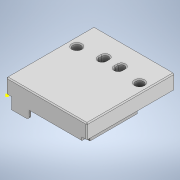
# Autodesk Inventor part: Cover_top
Saved by Autodesk Inventor 2022 (Build 260153000, 153)
## iProperties
Created: 2021-08-03
Part Number: Cover_top
Material: Generic
Document SubType Name: Modeling
Designer: exllu
Density: 1 g/cm^3
Appearance: Default
Author: exllu
Autodesk Inventor part; units mm, degrees
ref_plane "YZ Plane" through (0, 0, 0) normal (1, 0, 0) x (0, 1, 0)
ref_plane "XZ Plane" through (0, 0, 0) normal (0, 1, 0) x (-1, 0, 0)
ref_plane "XY Plane" through (0, 0, 0) normal (0, 0, 1) x (1, 0, 0)
sketch "Sketch1" plane through (0, 0, 0) normal (0, 1, 0) x (-1, 0, 0)
  line L0 (0, 0) -> (-80, 0)
  line L1 (-80, 0) -> (-80, -83)
  line L2 (-80, -83) -> (0, -83)
  line L3 (0, -83) -> (0, 0)
  dimension "d0" = 80
  dimension "d1" = 83
  constraints: 8 end point, 2 parallel, 1 horizontal, 1 perpendicular
  measures "d0" distance of L2.end L1.end
  measures "d1" distance of L1.end L0.end
extrude "Extrusion1" add sketch "Sketch1" along normal blind 16.25
sketch "Sketch2" plane through (0, 0, 0) normal (0, -1, 0) x (1, 0, 0)
  line L0 (0, -83) -> (0, 0) projected
  line L1 (0, 0) -> (0, -83)
  line L2 (80, -83) -> (0, -83) projected
  line L3 (80, 0) -> (80, -83) projected
  line L4 (0, -83) -> (80, -83)
  line L5 (80, -83) -> (80, -49.5)
  line L6 (80, -49.5) -> (0, -49.5)
  line L7 (0, -49.5) -> (0, -83)
  line L8 (80, -49.5) -> (0, -49.5)
  line L9 (0, -49.5) -> (0, 0)
  line L10 (0, 0) -> (80, 0)
  line L11 (80, 0) -> (80, -49.5)
  dimension "d4" = 33.5
  constraints: 18 end point, 4 parallel, 2 horizontal, 2 perpendicular, 1 point on line, 1 vertical
  measures "d4" distance of L5.end L4.end
extrude "Extrusion3" cut sketch "Sketch2" against normal blind 4 contours L0 L10 L3 L6
sketch "Sketch3" plane through (0, 4, 0) normal (0, -1, 0) x (1, 0, 0)
  line L0 (0, -83) -> (0, 0) projected
  line L1 (80, -49.5) -> (0, -49.5) projected
  line L2 (0, 0) -> (80, 0)
  line L3 (80, 0) -> (80, -49.5)
  line L4 (80, -49.5) -> (0, -49.5)
  line L5 (0, -49.5) -> (0, 0)
  constraints: 8 end point, 2 parallel, 1 horizontal, 1 perpendicular
extrude "Extrusion4" add sketch "Sketch3" along normal blind 13.169
sketch "Sketch4" plane through (0, 16.25, 0) normal (0, 0, 1) x (1, 0, 0)
  line L0 (80, 0) -> (0, 0) projected
  line L1 (0, 0) -> (80, 0)
  line L2 (80, -25.419) -> (80, 0) projected
  line L3 (80, 0) -> (80, -25.419)
  line L4 (80, -25.419) -> (38, -25.419)
  line L5 (80, -25.419) -> (0, -25.419) projected
  line L6 (38, -25.419) -> (38, -17)
  line L7 (38, -17) -> (80, -17)
  line L8 (80, -25.419) -> (77.5, -25.419)
  line L9 (77.5, -25.419) -> (77.5, -17)
  line L10 (77.5, -17) -> (80, -17)
  line L11 (77.5, -25.419) -> (75, -25.419)
  line L12 (75, -25.419) -> (75, -17)
  line L13 (75, -17) -> (77.5, -17)
  line L14 (77.5, -17) -> (77.5, -25.419)
  point P0 (0, -16.25)
  dimension "d11" = 42
  dimension "d12" = 8.419
  dimension "d13" = 2.5
  dimension "d14" = 2.5
  constraints: 24 end point, 6 perpendicular, 5 point on line, 2 horizontal, 2 parallel
  measures "d11" distance of L2.start L4.end
  measures "d12" distance of L4.end L6.end
  measures "d13" distance of L2.start L8.end
  measures "d14" distance of L12.end L13.end
extrude "Extrusion5" cut sketch "Sketch4" against normal blind 50 contours L4 L9 L7 L2 | L4 L6 L7 L12
sketch "Sketch5" plane through (77.5, -0.75, 0) normal (0, -1, 0) x (1, 0, 0)
  line L0 (-77.5, 0) -> (2.5, 0) projected
  line L1 (0, -49.5) -> (0, 0) projected
  line L2 (2.5, 0) -> (0, 0)
  line L3 (0, 0) -> (0, -49.5)
  line L4 (0, -49.5) -> (2.5, -49.5)
  line L5 (2.5, -49.5) -> (2.5, 0)
  constraints: 8 end point, 2 parallel, 1 horizontal, 1 perpendicular
extrude "Extrusion6" cut sketch "Sketch5" against normal blind 4.249
sketch "Sketch6" plane through (0, -9.169, 0) normal (0, -1, 0) x (1, 0, 0)
  line L0 (77.5, -49.5) -> (77.5, 0) projected
  line L1 (75, 0) -> (75, -49.5) projected
  line L2 (77.5, 0) -> (75, 0)
  line L3 (75, 0) -> (75, -2)
  line L4 (75, -2) -> (77.5, -2)
  line L5 (77.5, -2) -> (77.5, 0)
  point P0 (0, 0)
  dimension "d19" = 2
  constraints: 8 end point, 2 parallel, 1 horizontal, 1 perpendicular, 1 point on line
  measures "d19" distance of L3.end L2.end
extrude "Extrusion7" cut sketch "Sketch6" against normal blind 12.668
ref_plane "Work Plane1" through (40, 0, -83) normal (1, 0, 0) x (0, 0, -1)
mirror "Mirror1" about plane through (40, 0, -83) normal (1, 0, 0) of "Extrusion7", "Extrusion6"
sketch "Sketch7" plane through (0, -0.75, 0) normal (0, 0, 1) x (1, 0, 0)
  line L0 (0, 0) -> (0, -8.419) projected
  line L1 (2.5, -8.419) -> (0, -8.419) projected
  line L2 (0, 0) -> (2.5, 0)
  line L3 (2.5, 0) -> (2.5, -8.419)
  line L4 (2.5, -8.419) -> (0, -8.419)
  line L5 (0, -8.419) -> (0, 0)
  point P0 (0, 0.75)
  constraints: 8 end point, 2 parallel, 1 horizontal, 1 perpendicular
extrude "Extrusion8" cut sketch "Sketch7" against normal blind 50
sketch "Sketch8" plane through (0, -9.169, 0) normal (0, -1, 0) x (1, 0, 0)
  line L0 (2.5, -2) -> (5, -2) projected
  line L1 (75, -49.5) -> (38, -49.5) projected
  line L2 (5, -2) -> (75, -2)
  line L3 (75, -2) -> (75, -49.5)
  line L4 (75, -49.5) -> (5, -49.5)
  line L5 (5, -49.5) -> (5, -2)
  point P0 (0, 0)
  constraints: 8 end point, 2 parallel, 1 horizontal, 1 perpendicular
extrude "Extrusion9" cut sketch "Sketch8" against normal blind 22.419
sketch "Sketch10" plane through (0, 0, -83) normal (-1, 0, 0) x (0, 0, 1)
  line L0 (0, 0) -> (0, 16.25) projected
  line L1 (33.5, 0) -> (33.5, 13.25) projected
  line L2 (0, 0) -> (33.5, 0)
  line L3 (33.5, 0) -> (33.5, 3.5)
  line L4 (33.5, 3.5) -> (0, 3.5)
  line L5 (0, 3.5) -> (0, 0)
  point P0 (83, 0)
  dimension "d30" = 3.5
  constraints: 8 end point, 2 parallel, 1 horizontal, 1 perpendicular, 1 point on line
  measures "d30" distance of L3.end L2.end
extrude "Extrusion11" cut sketch "Sketch10" against normal blind 5.5
mirror "Mirror2" about plane through (40, 0, -83) normal (1, 0, 0) of "Extrusion11"
sketch "Sketch11" plane through (80, 16.25, -83) normal (0, 0, -1) x (-1, 0, 0)
  line L0 (80, -16.25) -> (64.5, -16.25)
  line L1 (5.5, -16.25) -> (74.5, -16.25) projected
  line L2 (64.5, -16.25) -> (64.5, -12.75)
  line L3 (64.5, -16.25) -> (68, -16.25) construction
  line L4 (74.5, -12.75) -> (80, -12.75) projected
  line L5 (64.5, -12.75) -> (74.5, -12.75)
  line L6 (74.5, -16.25) -> (74.5, -12.75) projected
  line L7 (74.5, -12.75) -> (74.5, -16.25)
  dimension "d33" = 15.5
  dimension "d34" = 3.5
  dimension "d35" = 90
  constraints: 10 end point, 2 perpendicular, 1 collinear, 1 horizontal, 1 point on line
  measures "d33" distance of L0.start L0.end
  measures "d34" distance of L0.end L2.end
  measures "d35" angle of L3 L2
extrude "Extrusion12" cut sketch "Sketch11" against normal blind 3.5
sketch "Sketch12" plane through (74.5, 3.5, -83) normal (0, -1, 0) x (1, 0, 0)
  line L0 (0, 0) -> (-59, 0) projected
  line L1 (5.5, 83) -> (5.5, 0) projected
  line L2 (0, 0) -> (5.5, 0)
  line L3 (5.5, 0) -> (5.5, 2.5)
  line L4 (5.5, 2.5) -> (0, 2.5)
  line L5 (0, 2.5) -> (0, 0)
  point P0 (-74.5, 83)
  dimension "d38" = 2.5
  constraints: 8 end point, 2 parallel, 1 horizontal, 1 perpendicular, 1 point on line
  measures "d38" distance of L3.end L2.end
extrude "Extrusion13" add sketch "Sketch12" along normal blind 3.5
sketch "Sketch13" plane through (0, 0, 0) normal (0, -1, 0) x (1, 0, 0)
  line L0 (80, 0) -> (80, -83) projected
  line L1 (80, -83) -> (65, -83)
  line L2 (65, -83) -> (65, -80.5)
  line L3 (65, -80.5) -> (80, -80.5)
  line L4 (80, -80.5) -> (80, -83)
  point P0 (0, 0)
  dimension "d41" = 15
  dimension "d42" = 2.5
  constraints: 8 end point, 2 parallel, 1 horizontal, 1 perpendicular
  measures "d41" distance of L2.end L3.end
  measures "d42" distance of L1.end L2.end
extrude "Extrusion14" add sketch "Sketch13" along normal blind 16.831
sketch "Sketch15" plane through (0, 16.25, 0) normal (0, 1, 0) x (1, 0, 0)
  line L0 (0, 0) -> (0, 83)
  line L1 (65, 83) -> (15.5, 83) projected
  line L2 (0, 83) -> (80, 83)
  line L3 (40, 83) -> (40, 60)
  line L4 (40, 60) -> (48, 60)
  line L5 (48, 60) -> (32, 60)
  circle A0 centre (32, 60) radius 1.75
  circle A1 centre (48, 60) radius 1.75
  dimension "d55" = 83
  dimension "d57" = 80
  dimension "d58" = 23
  dimension "d59" = 8
  dimension "d60" = 16
  dimension "d61" = 3.5
  dimension "d62" = 3.5
  constraints: 10 end point, 2 centre point, 2 coincident, 2 point on line, 2 vertical, 1 horizontal, 1 midpoint
  measures "d55" distance of L0.start L0.end
  measures "d57" distance of L0.end L2.end
  measures "d58" distance of L3.start L3.end
  measures "d59" distance of L3.end L4.end
  measures "d60" distance of L4.end L5.end
  measures "d61" diameter of A0
  measures "d62" diameter of A1
extrude "Extrusion16" cut sketch "Sketch15" against normal blind 50
sketch "Sketch16" plane through (0, 16.25, 0) normal (0, 1, 0) x (1, 0, 0)
  circle A0 centre (32, 60) radius 1.75 projected
  circle A1 centre (32, 60) radius 4
  circle A2 centre (48, 60) radius 1.75 projected
  circle A3 centre (48, 60) radius 4
  point P0 (0, 0)
  dimension "d65" = 8
  dimension "d66" = 8
  constraints: 2 centre point, 2 coincident
  measures "d65" diameter of A1
  measures "d66" diameter of A3
extrude "Extrusion17" cut sketch "Sketch16" against normal blind 10
sketch "Sketch19" plane through (0, 0, 0) normal (0, -1, 0) x (1, 0, 0)
  line L0 (74.5, -80.5) -> (74.5, -49.5) projected
  line L1 (15.5, -79.5) -> (5.5, -79.5) projected
  line L2 (74.5, -49.5) -> (5.5, -49.5)
  line L3 (5.5, -49.5) -> (5.5, -79.5)
  line L4 (5.5, -79.5) -> (15.5, -79.5)
  line L5 (74.5, -79.5) -> (74.5, -49.5)
  line L6 (15.5, -83) -> (15.5, -79.5) projected
  line L7 (65, -80.5) -> (65, -83) projected
  line L8 (15.5, -79.5) -> (65, -79.5)
  line L9 (65, -80.5) -> (65, -83)
  line L10 (65, -83) -> (15.5, -83)
  line L11 (15.5, -83) -> (15.5, -79.5)
  line L12 (65, -80.5) -> (74.5, -80.5) projected
  line L13 (74.5, -79.5) -> (65, -79.5)
  line L14 (65, -79.5) -> (65, -80.5)
  line L15 (65, -80.5) -> (74.5, -80.5)
  line L16 (74.5, -80.5) -> (74.5, -79.5)
  point P0 (0, 0)
  constraints: 24 end point, 6 parallel, 3 horizontal, 3 perpendicular, 2 point on line
extrude "Extrusion20" cut sketch "Sketch19" against normal blind 1.25
sketch "Sketch20" plane through (0, -9.169, 0) normal (0, -1, 0) x (1, 0, 0)
  line L0 (0, -49.5) -> (5, -49.5) projected
  line L1 (2.5, -2) -> (2.5, -49.5) projected
  line L2 (5, -49.5) -> (2.5, -49.5)
  line L3 (2.5, -49.5) -> (2.5, -2)
  line L4 (2.5, -2) -> (5, -2)
  line L5 (5, -2) -> (5, -49.5)
  line L6 (5, -2) -> (2.5, -2) projected
  line L7 (5, -2) -> (5.9402, -2)
  line L8 (5.9402, -2) -> (5.9402, -3.7491)
  line L9 (5.9402, -3.7491) -> (5, -3.7491)
  line L10 (5, -3.7491) -> (5, -2)
  point P0 (0, 0)
  constraints: 16 end point, 4 parallel, 2 horizontal, 2 perpendicular
extrude "Extrusion21" cut sketch "Sketch20" against normal blind 6
mirror "Mirror5" about plane through (40, 0, -83) normal (1, 0, 0) of "Extrusion21"
sketch "Sketch21" plane through (77.5, 3.499, -2) normal (1, 0, 0) x (0, 0, -1)
  line L0 (0, -6.668) -> (0, 0) projected
  line L1 (0, -6.668) -> (47.5, -6.668) projected
  line L2 (0, 0) -> (47.5, 0)
  line L3 (47.5, 0) -> (47.5, -6.668)
  line L4 (47.5, -6.668) -> (0, -6.668)
  line L5 (0, -6.668) -> (0, 0)
  point P0 (-2, -3.499)
  point P1 (1, -6.668)
  constraints: 8 end point, 2 parallel, 1 horizontal, 1 perpendicular
extrude "Extrusion22" cut sketch "Sketch21" against normal blind 0.5
mirror "Mirror6" about plane through (40, 0, -83) normal (1, 0, 0) of "Extrusion22"
sketch "Sketch22" plane through (5, -3.169, -2) normal (0, 0, 1) x (1, 0, 0)
  line L0 (0, 0) -> (-2, 0) projected
  line L1 (-5, 6.668) -> (0, 6.668) projected
  line L2 (0, 0) -> (-2, 0)
  line L3 (-2, 0) -> (-2, 6.668)
  line L4 (-2, 6.668) -> (0, 6.668)
  line L5 (0, 6.668) -> (0, 0)
  point P0 (-5, 3.169)
  point P1 (-4, 6.668)
  constraints: 8 end point, 2 parallel, 1 horizontal, 1 perpendicular, 1 point on line
extrude "Extrusion23" cut sketch "Sketch22" against normal blind 1
mirror "Mirror7" about plane through (40, 0, -83) normal (1, 0, 0) of "Extrusion23"
sketch "Sketch23" plane through (0, 16.25, 0) normal (0, 1, 0) x (1, 0, 0)
  circle A0 centre (32, 60) radius 4 projected
  arc A1 (36, 60) -> (28, 60) centre (32, 60) ccw
  line L0 (32, 60) -> (32, 57)
  arc A2 (28, 57) -> (36, 57) centre (32, 57) ccw
  line L1 (28, 57) -> (28, 60)
  line L2 (36, 60) -> (36, 57)
  line L3 (79, 83) -> (1, 83) projected
  line L4 (1, 83) -> (79, 83)
  line L5 (1, 83) -> (40, 83)
  line L6 (40, 83) -> (40, 30.6783)
  line L7 (65, 83) -> (80, 83) projected
  circle A3 centre (48, 60) radius 4
  arc A4 (52, 60) -> (44, 60) centre (48, 60) ccw
  line L8 (48, 60) -> (48, 57)
  arc A5 (44, 57) -> (52, 57) centre (48, 57) ccw
  line L9 (52, 57) -> (52, 60)
  line L10 (44, 60) -> (44, 57)
  point P0 (0, 0)
  point P1 (52, 60)
  point P2 (44, 60)
  dimension "d87" = 8
  dimension "d88" = 3
  dimension "d89" = 8
  dimension "d90" = 39
  constraints: 18 end point, 8 point on circle, 8 symmetric about line, 5 centre point, 4 coincident, 3 tangent, 1 collinear, 1 midpoint, 1 perpendicular, 1 vertical, 3 other
  measures "d87" diameter of A1
  measures "d88" distance of L0.start L0.end
  measures "d89" diameter of A2
  measures "d90" distance of L3.end L5.end
sketch "Sketch24" plane through (0, 6.25, 0) normal (0, 1, 0) x (1, 0, 0)
  arc A0 (33.75, 60) -> (30.25, 60) centre (32, 60) ccw
  circle A1 centre (48, 60) radius 1.75 projected
  arc A2 (49.75, 60) -> (46.25, 60) centre (48, 60) ccw
  line L0 (48, 60) -> (48, 57)
  arc A3 (46.25, 57) -> (49.75, 57) centre (48, 57) ccw
  line L1 (46.25, 57) -> (46.25, 60)
  line L2 (49.75, 60) -> (49.75, 57)
  circle A4 centre (32, 60) radius 1.75 projected
  line L3 (32, 60) -> (32, 63)
  arc A5 (36, 63) -> (28, 63) centre (32, 63) ccw
  circle A6 centre (32, 60) radius 4 projected
  line L4 (28, 60) -> (28, 63)
  line L5 (36, 63) -> (36, 60)
  arc A7 (28, 60) -> (36, 60) centre (32, 60) ccw
  line L6 (32, 60) -> (48, 60)
  line L7 (40, 60) -> (40, 64.9019)
  arc A8 (52, 63) -> (44, 63) centre (48, 63) ccw
  line L8 (52, 60) -> (52, 63)
  line L9 (44, 63) -> (44, 60)
  arc A9 (44, 60) -> (52, 60) centre (48, 60) ccw
  point P0 (0, 0)
  point P1 (49.75, 60)
  point P2 (46.25, 60)
  point P3 (49.6223, 56.3437)
  point P4 (46.25, 60)
  dimension "d93" = 3.5
  dimension "d94" = 3.5
  dimension "d96" = 3
  dimension "d98" = 3.5
  dimension "d107" = 3
  dimension "d108" = 8
  constraints: 20 end point, 16 point on circle, 7 centre point, 6 symmetric about line, 6 tangent, 5 coincident, 3 vertical, 1 horizontal, 1 midpoint, 2 other
  measures "d93" diameter of A0
  measures "d94" diameter of A2
  measures "d96" distance of L0.start L0.end
  measures "d98" diameter of A3
  measures "d107" distance of L3.start L3.end
  measures "d108" diameter of A5
sketch "Sketch25" plane through (0, 1.25, 0) normal (0, -1, 0) x (1, 0, 0)
  line L0 (0, -49.5) -> (5, -49.5) projected
  line L1 (0, 0) -> (0, -49.5)
  line L2 (5.5, -49.5) -> (74.5, -49.5) projected
  line L3 (0, -49.5) -> (5.5, -49.5)
  line L4 (5.5, -79.5) -> (5.5, -49.5) projected
  circle A0 centre (71, -55) radius 4 projected
  line L5 (5.5, -49.5) -> (74.1225, -49.5)
  line L6 (74.1225, -49.5) -> (74.1225, -52.5)
  line L7 (74.1225, -52.5) -> (5.5, -52.5)
  line L8 (5.5, -52.5) -> (5.5, -49.5)
  dimension "d104" = 3
  constraints: 12 end point, 2 parallel, 1 collinear, 1 horizontal, 1 perpendicular, 1 vertical, 2 other
  measures "d104" distance of L5.end L6.end
extrude "Extrusion26" cut sketch "Sketch25" against normal blind 12 contours L2 L6 A0 L7 L4 | L7 A0 picked at (71, -52)
extrude "Extrusion27" cut sketch "Sketch24" along normal blind 12 contours A1 L6 L9 A8 L8 A9 A3 L2 | L5 A6 L4 A5
sketch "Sketch26" plane through (0, 6.25, 0) normal (0, 1, 0) x (1, 0, 0)
  circle A0 centre (32, 60) radius 1.75 projected
  line L0 (32, 60) -> (32, 63)
  circle A1 centre (48, 60) radius 1.75 projected
  line L1 (48, 60) -> (48, 63)
  circle A2 centre (48, 63) radius 1.75
  arc A3 (33.75, 63) -> (30.25, 63) centre (32, 63) ccw
  line L2 (30.25, 63) -> (30.25, 60)
  line L3 (46.25, 63) -> (46.25, 60)
  line L4 (33.75, 63) -> (33.75, 60)
  arc A4 (30.25, 60) -> (33.75, 60) centre (32, 60) ccw
  line L5 (32, 60) -> (48, 60)
  line L6 (40, 60) -> (40, 64.1787)
  circle A5 centre (48, 60) radius 1.75
  arc A6 (49.75, 63) -> (46.25, 63) centre (48, 63) ccw
  line L7 (49.75, 63) -> (49.75, 60)
  line L8 (46.25, 63) -> (46.25, 60)
  point P0 (0, 0)
  point P1 (47.0986, 61.5)
  point P2 (48.9014, 61.5)
  point P3 (49.75, 60)
  dimension "d113" = 3.5
  dimension "d111" = 3
  dimension "d112" = 3
  dimension "d114" = 3.5
  constraints: 18 end point, 10 point on circle, 4 centre point, 4 symmetric about line, 4 tangent, 4 vertical, 3 coincident, 1 midpoint, 1 perpendicular, 7 other
  measures "d111" distance of L0.start L0.end
  measures "d112" distance of L1.start L1.end
  measures "d114" diameter of A3
extrude "Extrusion28" cut sketch "Sketch26" against normal blind 12 contours L2 A3 L4 A0 | L3 A2 A1 | A1 A2 L7 | A2 A1 | A1 L1 A2 | A2 L1 A1
sketch "Sketch29" plane through (0, 16.25, 0) normal (0, 1, 0) x (1, 0, 0)
  arc A0 (72.75, 58) -> (69.25, 58) centre (71, 58) ccw projected
  circle A1 centre (71, 58) radius 1.75
  point P0 (0, 0)
  constraints: 1 centre point, 1 coincident
extrude "Extrusion30" cut sketch "Sketch29" against normal blind 30
sketch "Sketch30" plane through (0, 16.25, 0) normal (0, 1, 0) x (1, 0, 0)
  circle A0 centre (71, 58) radius 1.75 projected
  circle A1 centre (71, 58) radius 4
  point P0 (0, 0)
  dimension "d129" = 8
  constraints: 1 centre point, 1 coincident
  measures "d129" diameter of A1
extrude "Extrusion31" cut sketch "Sketch30" against normal blind 12 contours A0 | A1
mirror "Mirror8" about plane through (40, 0, -83) normal (1, 0, 0) of "Extrusion30", "Extrusion31"
sketch "Sketch31" plane through (74.5, 3.5, -49.5) normal (1, 0, 0) x (0, 0, -1)
  line L0 (3, 0) -> (0, 0) projected
  line L1 (3, -2.25) -> (3, 0) projected
  line L2 (0, 0) -> (3, 0)
  line L3 (3, 0) -> (3, -2.25)
  line L4 (3, -2.25) -> (0, -2.25)
  line L5 (0, -2.25) -> (0, 0)
  point P0 (-49.5, -3.5)
  constraints: 8 end point, 2 parallel, 1 horizontal, 1 perpendicular
extrude "Extrusion32" cut sketch "Sketch31" against normal blind 100
sketch "Sketch32" plane through (0, 16.25, 0) normal (0, 0, 1) x (1, 0, 0)
  line L0 (0, -12.751) -> (0, 0) projected
  line L1 (80, -12.751) -> (80, 0) projected
  line L2 (0, 0) -> (80, 0)
  line L3 (80, 0) -> (80, -12.751)
  line L4 (80, -12.751) -> (75, -12.751)
  line L5 (75, -17) -> (75, -12.751) projected
  line L6 (75, -12.751) -> (75, -17)
  line L7 (38, -17) -> (75, -17) projected
  line L8 (75, -17) -> (38, -17)
  line L9 (38, -25.419) -> (5, -25.419) projected
  line L10 (38, -17) -> (38, -25.419)
  line L11 (38, -25.419) -> (5, -25.419)
  line L12 (5, -12.751) -> (5, -25.419) projected
  line L13 (5, -25.419) -> (5, -12.751)
  line L14 (0, -12.751) -> (5, -12.751) projected
  line L15 (5, -12.751) -> (0, -12.751)
  line L16 (0, -12.751) -> (0, 0)
  point P0 (0, -16.25)
  constraints: 20 end point, 5 perpendicular, 4 collinear, 1 horizontal
extrude "Extrusion33" add sketch "Sketch32" along normal blind 2
sketch "Sketch33" plane through (38, -9.169, -2) normal (0, 0, -1) x (-1, 0, 0)
  line L0 (0, 0) -> (0, 8.419) projected
  line L1 (33, 0) -> (0, 0) projected
  line L2 (0, 0) -> (33, 0)
  line L3 (33, 12.668) -> (33, 22.419) projected
  line L4 (33, 0) -> (33, 22.419)
  line L5 (33, 22.419) -> (-37, 22.419) projected
  line L6 (33, 22.419) -> (-37, 22.419)
  line L7 (-37, 8.419) -> (-37, 12.668) projected
  line L8 (-37, 22.419) -> (-37, 8.419)
  line L9 (0, 8.419) -> (-37, 8.419) projected
  line L10 (-37, 8.419) -> (0, 8.419)
  line L11 (0, 8.419) -> (0, 0)
  point P0 (38, 9.169)
  constraints: 12 end point, 3 collinear, 2 perpendicular, 1 horizontal
extrude "Extrusion34" cut sketch "Sketch33" against normal blind 2
sketch "Sketch35" plane through (74.1225, 3.5, -49.5) normal (-1, 0, 0) x (0, 0, 1)
  line L0 (0, -6.669) -> (0, 0) projected
  line L1 (-3, -2.25) -> (-3, 9.75) projected
  line L2 (0, 0) -> (-3, 0)
  line L3 (-3, 0) -> (-3, 9.75)
  line L4 (-3, 9.75) -> (0, 9.75)
  line L5 (0, 9.75) -> (0, 0)
  point P0 (49.5, -3.5)
  point P1 (-3, 0)
  point P2 (-3, 0)
  constraints: 8 end point, 2 parallel, 1 horizontal, 1 perpendicular
extrude "Extrusion36" cut sketch "Sketch35" against normal blind 0.878
sketch "Sketch36" plane through (5.5, 3.5, -52.5) normal (1, 0, 0) x (0, 0, -1)
  line L0 (0, 0) -> (-3, 0) projected
  line L1 (0, 0) -> (-3, 0)
  line L2 (-3, 0) -> (-3, 9.75)
  line L3 (-3, 9.75) -> (0, 9.75)
  line L4 (0, 9.75) -> (0, 0)
  point P0 (-52.5, -3.5)
  constraints: 8 end point, 2 parallel, 1 horizontal, 1 perpendicular
extrude "Extrusion37" cut sketch "Sketch36" against normal blind 0.5
sketch "Sketch37" plane through (0, 3.5, -83) normal (0, -1, 0) x (1, 0, 0)
  line L0 (80, 0) -> (0, 0) projected
  line L1 (15.5, 3.5) -> (5.5, 3.5) projected
  line L2 (0, 0) -> (15.5, 0)
  line L3 (15.5, 0) -> (15.5, 3.5)
  line L4 (15.5, 3.5) -> (0, 3.5)
  line L5 (0, 3.5) -> (0, 0)
  line L6 (0, 0) -> (5.5, 0)
  line L7 (5.5, 0) -> (5.5, 30.5)
  line L8 (5.5, 30.5) -> (0, 30.5)
  line L9 (0, 30.5) -> (0, 0)
  line L10 (5, 33.5) -> (3, 33.5) projected
  line L11 (0, 30.5) -> (5, 30.5)
  line L12 (5, 30.5) -> (5, 33.5)
  line L13 (5, 33.5) -> (0, 33.5)
  line L14 (0, 33.5) -> (0, 30.5)
  line L15 (0, 33.5) -> (0, 85) projected
  line L16 (0, 33.5) -> (0, 85)
  line L17 (0, 85) -> (5, 85)
  line L18 (80, 85) -> (0, 85) projected
  line L19 (5, 83) -> (5, 80) projected
  line L20 (5, 80) -> (5, 85)
  line L21 (3, 80) -> (5, 80) projected
  line L22 (5, 80) -> (3, 80)
  line L23 (3, 80) -> (3, 33.5) projected
  line L24 (3, 80) -> (3, 33.5)
  point P0 (0, 83)
  constraints: 34 end point, 6 parallel, 3 collinear, 3 horizontal, 3 perpendicular, 1 point on line, 1 vertical
extrude "Extrusion38" add sketch "Sketch37" along normal blind 1.25
sketch "Sketch38" plane through (74.5, 3.5, -80.5) normal (0, -1, 0) x (1, 0, 0)
  line L0 (5.5, 0) -> (-9.5, 0) projected
  line L1 (5.5, 82.5) -> (5.5, 31) projected
  line L2 (5.5, 0) -> (5.5, 82.5)
  line L3 (5.5, 82.5) -> (0.5, 82.5)
  line L4 (0.5, 82.5) -> (0.5, 77.5)
  line L5 (0.5, 80.5) -> (0.5, 31) projected
  line L6 (2.5, 77.5) -> (2.5, 31) projected
  line L7 (0.5, 77.5) -> (2.5, 77.5)
  line L8 (2.5, 77.5) -> (2.5, 31)
  line L9 (2.5, 31) -> (0.5, 31)
  line L10 (0.5, 31) -> (0.5, 28)
  line L11 (0.5, 28) -> (0, 28)
  line L12 (0.5005, 28) -> (-69.5, 28) projected
  line L13 (0, 28) -> (0, 0)
  line L14 (0, 0) -> (5.5, 0)
  point P0 (-74.5, 80.5)
  point P1 (0, 0)
  dimension "d151" = 5
  dimension "d152" = 0.5
  constraints: 20 end point, 4 perpendicular, 4 point on line, 2 collinear
  measures "d151" distance of L3.end L4.end
  measures "d152" distance of L10.end L11.end
extrude "Extrusion39" add sketch "Sketch38" along normal blind 1.25 contours L0 L13 L11 L10 L9 L6 L7 L4 L3 L1 L2
sketch "Sketch39" plane through (0, 1.25, 0) normal (0, -1, 0) x (1, 0, 0)
  line L0 (74.5, -80.5) -> (74.5, -52.5) projected
  line L1 (5.5, -52.5) -> (5.5, -79.5) projected
  line L2 (74.5, -80.5) -> (5.5, -80.5)
  line L3 (5.5, -80.5) -> (5.5, -52.5)
  line L4 (5.5, -52.5) -> (74.5, -52.5)
  line L5 (74.5, -52.5) -> (74.5, -80.5)
  line L6 (5.5, -79.5) -> (5.5, -52.5) projected
  line L7 (15.5, -83) -> (15.5, -79.5) projected
  line L8 (5.5, -79.5) -> (15.5, -79.5)
  line L9 (15.5, -79.5) -> (15.5, -80.5)
  line L10 (15.5, -80.5) -> (5.5, -80.5)
  line L11 (5.5, -80.5) -> (5.5, -79.5)
  line L12 (74.5, -80.5) -> (65, -80.5) projected
  line L13 (15.5, -83) -> (65, -83)
  line L14 (65, -83) -> (65, -80.5)
  line L15 (65, -80.5) -> (15.5, -80.5)
  line L16 (15.5, -80.5) -> (15.5, -83)
  point P0 (0, 0)
  constraints: 24 end point, 6 parallel, 3 horizontal, 3 perpendicular, 2 point on line
extrude "Extrusion40" add sketch "Sketch39" along normal blind 1.25 contours L2 L7 L8 L1 L4 L0 | L14 L13 L7 L2
sketch "Sketch40" plane through (0, 16.25, 0) normal (0, 1, 0) x (1, 0, 0)
  circle A0 centre (9, 58) radius 1.75 projected
  circle A1 centre (9, 58) radius 1.75
  circle A2 centre (9, 58) radius 4
  arc A3 (30.25, 60) -> (33.75, 60) centre (32, 60) ccw projected
  arc A4 (30.25, 60) -> (33.75, 60) centre (32, 60) ccw
  arc A5 (33.75, 63) -> (30.25, 63) centre (32, 63) ccw projected
  arc A6 (33.75, 63) -> (30.3777, 63.6563) centre (32, 63) ccw
  arc A7 (28, 60) -> (36, 60) centre (32, 60) ccw projected
  line L0 (36, 60) -> (36, 63)
  line L1 (33.75, 60) -> (33.75, 63) projected
  line L2 (33.75, 63) -> (33.75, 60)
  arc A8 (36, 63) -> (33.75, 66.5969) centre (32, 63) ccw
  arc A9 (28, 60) -> (36, 60) centre (32, 60) ccw
  arc A10 (36, 63) -> (28, 63) centre (32, 63) ccw
  line L3 (28, 60) -> (28, 63) projected
  line L4 (28, 60) -> (28, 63)
  line L5 (30.25, 63) -> (30.25, 60) projected
  line L6 (30.25, 60) -> (30.25, 63)
  arc A11 (46.25, 60) -> (49.75, 60) centre (48, 60) ccw projected
  line L7 (32, 60) -> (48, 60)
  line L8 (48, 60) -> (40, 60)
  line L9 (40, 60) -> (40, 47.3434)
  circle A12 centre (71, 58) radius 1.75
  circle A13 centre (71, 58) radius 1.75
  circle A14 centre (71, 58) radius 4
  arc A15 (46.25, 60) -> (49.75, 60) centre (48, 60) ccw
  arc A16 (46.25, 60) -> (49.75, 60) centre (48, 60) ccw
  arc A17 (49.75, 63) -> (46.25, 63) centre (48, 63) ccw
  arc A18 (49.6223, 63.6563) -> (46.25, 63) centre (48, 63) ccw
  arc A19 (44, 60) -> (52, 60) centre (48, 60) ccw
  line L10 (44, 60) -> (44, 63)
  line L11 (46.25, 60) -> (46.25, 63)
  line L12 (46.25, 63) -> (46.25, 60)
  arc A20 (46.25, 66.5969) -> (44, 63) centre (48, 63) ccw
  arc A21 (44, 60) -> (52, 60) centre (48, 60) ccw
  arc A22 (52, 63) -> (44, 63) centre (48, 63) ccw
  line L13 (52, 60) -> (52, 63)
  line L14 (52, 60) -> (52, 63)
  line L15 (49.75, 63) -> (49.75, 60)
  line L16 (49.75, 60) -> (49.75, 63)
  point P0 (0, 0)
  constraints: 30 point on circle, 28 end point, 23 symmetric about line, 18 centre point, 14 coincident, 4 point on line, 4 tangent, 2 collinear, 2 vertical, 1 horizontal, 1 midpoint, 11 other
extrude "Extrusion41" cut sketch "Sketch40" against normal blind 30 contours A0 | L5 A5 L1 A3 | L11 A17 L15 A11 | A12
sketch "Sketch41" plane through (0, 6.25, 0) normal (0, 1, 0) x (1, 0, 0)
  arc A0 (28, 60) -> (36, 60) centre (32, 60) ccw projected
  arc A1 (28, 60) -> (36, 60) centre (32, 60) ccw
  arc A2 (36, 63) -> (28, 63) centre (32, 63) ccw projected
  arc A3 (36, 63) -> (28, 63) centre (32, 63) ccw
  line L0 (28, 63) -> (28, 60) projected
  line L1 (28, 60) -> (28, 63)
  line L2 (36, 63) -> (37, 63) projected
  line L3 (36, 63) -> (36, 60)
  arc A4 (52, 63) -> (44, 63) centre (48, 63) ccw projected
  line L4 (32, 63) -> (48, 63)
  line L5 (40, 63) -> (40, 64.9814)
  arc A5 (44, 60) -> (52, 60) centre (48, 60) ccw
  arc A6 (44, 60) -> (52, 60) centre (48, 60) ccw
  arc A7 (52, 63) -> (44, 63) centre (48, 63) ccw
  arc A8 (52, 63) -> (44, 63) centre (48, 63) ccw
  line L6 (52, 63) -> (52, 60)
  line L7 (52, 60) -> (52, 63)
  line L8 (44, 63) -> (43, 63)
  line L9 (44, 63) -> (44, 60)
  line L10 (48, 63) -> (32, 63)
  point P0 (0, 0)
  constraints: 18 end point, 14 symmetric about line, 12 point on circle, 6 centre point, 6 point on line, 4 coincident, 1 collinear, 1 horizontal, 1 midpoint, 1 tangent, 1 vertical, 4 other
extrude "Extrusion42" cut sketch "Sketch41" against normal blind 4.25
sketch "Sketch42" plane through (65, -16.831, -80.5) normal (0, 0, 1) x (1, 0, 0)
  line L0 (0, 0) -> (0, 16.831) projected
  line L1 (15, 0) -> (0, 0) projected
  line L2 (0, 16.831) -> (15, 16.831)
  line L3 (15, 16.831) -> (15, 0)
  line L4 (15, 0) -> (0, 0)
  line L5 (0, 0) -> (0, 16.831)
  line L6 (15, 19.081) -> (9.5, 19.081) projected
  line L7 (9.5, 19.081) -> (15, 19.081)
  line L8 (15, 19.081) -> (15, 16.831)
  line L9 (15, 16.831) -> (9.5, 16.831)
  line L10 (9.5, 16.831) -> (9.5, 19.081)
  point P0 (-65, 16.831)
  constraints: 16 end point, 4 parallel, 2 horizontal, 2 perpendicular
extrude "Extrusion43" cut sketch "Sketch42" against normal blind 19.081
sketch "Sketch45" plane through (0, 0, 0) normal (0, -1, 0) x (1, 0, 0)
  point P0 (0, 0)
sketch "Sketch46" plane through (0, 0, 0) normal (0, -1, 0) x (1, 0, 0)
  line L0 (5.5, -79.5) -> (15.5, -79.5) projected
  line L1 (5.5, -79.5) -> (15.5, -79.5)
  line L2 (15.5, -79.5) -> (15.5, -83)
  line L3 (15.5, -83) -> (5.5, -83)
  line L4 (5.5, -83) -> (5.5, -79.5)
  point P0 (0, 0)
  constraints: 8 end point, 2 parallel, 1 horizontal, 1 perpendicular
extrude "Extrusion44" add sketch "Sketch46" against normal blind 10
sketch "Sketch47" plane through (0, 16.25, 2) normal (0, 0, 1) x (1, 0, 0)
  line L0 (38, -25.419) -> (38, -17) projected
  line L1 (5, -25.419) -> (38, -25.419) projected
  line L2 (38, -17) -> (23, -17)
  line L3 (23, -17) -> (23, -25.419)
  line L4 (23, -25.419) -> (38, -25.419)
  line L5 (38, -25.419) -> (38, -17)
  point P0 (0, -16.25)
  dimension "d174" = 15
  constraints: 8 end point, 2 parallel, 1 horizontal, 1 perpendicular, 1 point on line
  measures "d174" distance of L4.end L3.end
extrude "Extrusion45" cut sketch "Sketch47" against normal blind 10
sketch "Sketch48" plane through (5, -9.169, 0) normal (-1, 0, 0) x (0, 0, 1)
  line L0 (0, 8.419) -> (0, 11.419) projected
  line L1 (2, 11.419) -> (2, 0) projected
  line L2 (0, 11.419) -> (2, 11.419)
  line L3 (2, 11.419) -> (2, 0)
  line L4 (2, 0) -> (0, 0)
  line L5 (0, 0) -> (0, 11.419)
  point P0 (0, 9.169)
  point P1 (0, 8.419)
  constraints: 8 end point, 2 parallel, 1 horizontal, 1 perpendicular
extrude "Extrusion46" cut sketch "Sketch48" against normal blind 0.3
sketch "Sketch49" plane through (0, 2, 0) normal (0, 1, 0) x (1, 0, 0)
  arc A0 (46.25, 60) -> (49.75, 60) centre (48, 60) ccw projected
  arc A1 (46.6, 60) -> (49.4, 60) centre (48, 60) ccw
  arc A2 (49.75, 63) -> (46.25, 63) centre (48, 63) ccw projected
  arc A3 (49.4, 63) -> (46.6, 63) centre (48, 63) ccw
  arc A4 (30.25, 60) -> (33.75, 60) centre (32, 60) ccw projected
  arc A5 (30.6, 60) -> (33.4, 60) centre (32, 60) ccw
  arc A6 (33.75, 63) -> (30.25, 63) centre (32, 63) ccw projected
  arc A7 (33.4, 63) -> (30.6, 63) centre (32, 63) ccw
  arc A8 (36, 63) -> (28, 63) centre (32, 63) ccw
  arc A9 (28, 60) -> (36, 60) centre (32, 60) ccw
  line L0 (36, 63) -> (36, 60) projected
  line L1 (36, 63) -> (36, 60)
  line L2 (33.4, 63) -> (33.4, 60)
  line L3 (30.6, 60) -> (30.6, 63)
  arc A10 (36, 63) -> (28, 63) centre (32, 63) ccw projected
  line L4 (28, 60) -> (28, 63)
  arc A11 (52, 63) -> (44, 63) centre (48, 63) ccw projected
  arc A12 (52, 63) -> (44, 63) centre (48, 63) ccw
  arc A13 (44, 60) -> (52, 60) centre (48, 60) ccw projected
  arc A14 (44, 60) -> (52, 60) centre (48, 60) ccw
  line L5 (52, 63) -> (52, 60) projected
  line L6 (52, 60) -> (52, 63)
  line L7 (44, 60) -> (44, 63) projected
  line L8 (44, 60) -> (44, 63)
  line L9 (46.6, 60) -> (46.6, 63)
  line L10 (49.4, 60) -> (49.4, 63)
  point P0 (0, 0)
  dimension "d180" = 2.8
  dimension "d181" = 2.8
  dimension "d182" = 2.8
  dimension "d183" = 2.8
  constraints: 17 point on circle, 16 end point, 11 tangent, 8 centre point, 8 coincident, 6 point on line, 3 collinear, 1 vertical
  measures "d180" diameter of A1
  measures "d181" diameter of A3
  measures "d182" diameter of A5
  measures "d183" diameter of A7
extrude "Extrusion47" add sketch "Sketch49" along normal blind 8
sketch "Sketch50" plane through (0, 10, 0) normal (0, 1, 0) x (1, 0, 0)
  arc A0 (46.6, 60) -> (49.4, 60) centre (48, 60) ccw projected
  arc A1 (44.75, 60) -> (51.25, 60) centre (48, 60) ccw
  arc A2 (49.4, 63) -> (46.6, 63) centre (48, 63) ccw projected
  arc A3 (51.25, 63) -> (44.75, 63) centre (48, 63) ccw
  arc A4 (28, 60) -> (36, 60) centre (32, 60) ccw projected
  arc A5 (28.75, 60) -> (35.25, 60) centre (32, 60) ccw
  arc A6 (33.4, 63) -> (30.6, 63) centre (32, 63) ccw projected
  arc A7 (35.25, 63) -> (28.75, 63) centre (32, 63) ccw
  line L0 (37.4923, 70.7026) -> (25.239, 70.7026)
  line L1 (25.239, 70.7026) -> (25.239, 50.21)
  line L2 (25.239, 50.21) -> (37.4923, 50.21)
  line L3 (37.4923, 50.21) -> (37.4923, 70.7026)
  line L4 (54.0684, 71.4664) -> (42.3676, 71.4664)
  line L5 (42.3676, 71.4664) -> (42.3676, 49.9013)
  line L6 (42.3676, 49.9013) -> (54.0684, 49.9013)
  line L7 (54.0684, 49.9013) -> (54.0684, 71.4664)
  line L8 (35.25, 63) -> (35.25, 60)
  line L9 (28.75, 60) -> (28.75, 63)
  line L10 (44.75, 60) -> (44.75, 63)
  line L11 (51.25, 60) -> (51.25, 63)
  point P0 (0, 0)
  dimension "d186" = 6.5
  dimension "d187" = 6.5
  dimension "d188" = 6.5
  dimension "d189" = 6.5
  constraints: 24 end point, 8 point on circle, 5 tangent, 4 centre point, 4 coincident, 4 parallel, 2 horizontal, 2 perpendicular
  measures "d186" diameter of A1
  measures "d187" diameter of A3
  measures "d188" diameter of A5
  measures "d189" diameter of A7
extrude "Extrusion48" add sketch "Sketch50" along normal blind 6.25
chamfer "Chamfer9" distance 1 angle 45 10 edges at (67, 16.25, -58) (48, 16.25, -56.75) (44.75, 16.25, -61.5) (48, 16.25, -66.25) (51.25, 16.25, -61.5) (32, 16.25, -56.75) (28.75, 16.25, -61.5) (32, 16.25, -66.25) (35.25, 16.25, -61.5) (13, 16.25, -58)
sketch "Sketch52" plane through (0, 0, 0) normal (0, -1, 0) x (1, 0, 0)
  line L0 (74.5, -52.5) -> (74.5, -83) projected
  line L1 (5.5, -83) -> (5.5, -52.5) projected
  line L2 (74.5, -83) -> (5.5, -83)
  line L3 (5.5, -83) -> (5.5, -67)
  line L4 (5.5, -67) -> (74.5, -67)
  line L5 (74.5, -67) -> (74.5, -83)
  point P0 (0, 0)
  dimension "d195" = 16
  constraints: 8 end point, 2 parallel, 1 horizontal, 1 perpendicular, 1 point on line
  measures "d195" distance of L2.end L3.end
extrude "Extrusion49" cut sketch "Sketch52" against normal blind 10
chamfer "Chamfer10" distance 3 angle 45 1 edges at (40, 10, -67)
sketch "Sketch53" plane through (0, 16.25, 2) normal (0, 0, 1) x (1, 0, 0)
  point P0 (0, -16.25)
sketch "Sketch54" plane through (0, 16.25, 2) normal (0, 0, 1) x (1, 0, 0)
  line L0 (0, 0) -> (0, -14) projected
  line L1 (80, -14) -> (80, 0) projected
  line L2 (0, 0) -> (80, 0)
  line L3 (80, 0) -> (80, -14)
  line L4 (80, -14) -> (0, -14)
  line L5 (0, -14) -> (0, 0)
  line L6 (80, -14) -> (75, -14) projected
  line L7 (23, -17) -> (75, -17) projected
  line L8 (75, -14) -> (23, -14)
  line L9 (23, -14) -> (23, -17)
  line L10 (23, -17) -> (75, -17)
  line L11 (75, -17) -> (75, -14)
  line L12 (0, -14) -> (5.3, -14) projected
  line L13 (23, -17) -> (23, -25.419) projected
  line L14 (5.3, -14) -> (23, -14)
  line L15 (23, -14) -> (23, -25.419)
  line L16 (23, -25.419) -> (5.3, -25.419)
  line L17 (5.3, -25.419) -> (5.3, -14)
  point P0 (0, -16.25)
  point P1 (79, -14)
  point P2 (1, -14)
  constraints: 24 end point, 6 parallel, 3 horizontal, 3 perpendicular
extrude "Extrusion50" add sketch "Sketch54" along normal blind 1
sketch "Sketch55" plane through (38, -9.169, 0) normal (0, 0, -1) x (-1, 0, 0)
  line L0 (15, 8.419) -> (15, 0) projected
  line L1 (32.7, 0) -> (15, 0) projected
  line L2 (15, 8.419) -> (32.7, 8.419)
  line L3 (32.7, 8.419) -> (32.7, 0)
  line L4 (32.7, 0) -> (15, 0)
  line L5 (15, 0) -> (15, 8.419)
  point P0 (38, 9.169)
  constraints: 8 end point, 2 parallel, 1 horizontal, 1 perpendicular
extrude "Extrusion51" cut sketch "Sketch55" against normal blind 1.5
chamfer "Chamfer11" distance 1 angle 45 5 edges at (0, 16.25, -40) (40, 16.25, 3) (80, 16.25, -40) (80, 9.25, 3) (0, 9.25, 3)
fillet "Fillet2" radius 3 1 edges at (23, -9.169, 2.25)
sketch "Sketch57" plane through (0, 0, 0) normal (0, -1, 0) x (1, 0, 0)
  line L0 (74.5, -52.5) -> (74.5, -67) projected
  line L1 (5.5, -67) -> (74.5, -67)
  line L2 (74.5, -67) -> (74.5, -52.5)
  line L3 (74.5, -52.5) -> (5.5, -52.5)
  line L4 (5.5, -52.5) -> (5.5, -67)
  point P0 (0, 0)
  constraints: 8 end point, 2 parallel, 1 horizontal, 1 perpendicular
extrude "Extrusion52" cut sketch "Sketch57" against normal blind 1
body "Solid1"
